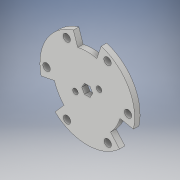
# Autodesk Inventor part: NewMechanumWheelHub
Saved by Autodesk Inventor 2017 (Build 210142000, 142)
## iProperties
Created: 2017-12-16
Part Number: NewMechanumWheelHub
Material: Generic
Document SubType Name: Modeling
Designer: User
Density: 1 g/cm^3
Appearance: Default
Author: User
Autodesk Inventor part; units mm, degrees
ref_plane "YZ Plane" through (0, 0, 0) normal (1, 0, 0) x (0, 1, 0)
ref_plane "XZ Plane" through (0, 0, 0) normal (0, 1, 0) x (-1, 0, 0)
ref_plane "XY Plane" through (0, 0, 0) normal (0, 0, 1) x (1, 0, 0)
sketch "Sketch1" plane through (0, 0, 0) normal (0, 0, 1) x (1, 0, 0)
  circle A0 centre (0, 0) radius 27.6352
  dimension "d0" = 55.2704
  constraints: 1 centre point, 1 coincident
  measures "d0" diameter of A0
extrude "Extrusion1" add sketch "Sketch1" along normal blind 3.175
sketch "Sketch2" plane through (0, 0, 3.175) normal (0, 0, 1) x (1, 0, 0)
  circle A0 centre (0, 0) radius 27.6352 projected
  line L0 (0, 27.6352) -> (0, 0)
  line L1 (0, 0) -> (23.9328, -13.8176)
  line L2 (0, 0) -> (-23.9328, -13.8176)
  line L3 (0, 0) -> (27.6352, 0) construction
  line L4 (0, 27.6352) -> (0, 19.4152)
  line L5 (0, 19.4152) -> (5.08, 19.4152)
  line L6 (0, 19.4152) -> (-5.08, 19.4152)
  arc A1 (5.08, 19.4152) -> (-5.08, 19.4152) centre (0, -5.5937) ccw
  line L7 (-5.08, 19.4152) -> (2.5298, 19.4152) construction
  line L8 (-5.08, 19.4152) -> (-7.5281, 26.5901)
  line L9 (-5.08, 19.4152) -> (2.501, 19.4152) construction
  line L10 (5.08, 19.4152) -> (7.5281, 26.5901)
  line L11 (5.08, 19.4152) -> (12.661, 19.4152) construction
  line L12 (23.9328, -13.8176) -> (16.8277, -9.7155)
  line L13 (16.8277, -9.7155) -> (19.355, -5.3381)
  line L14 (16.8277, -9.7155) -> (14.3004, -14.0929)
  line L15 (16.8277, -9.7155) -> (17.2897, -9.9822)
  arc A2 (14.3004, -14.0929) -> (19.355, -5.3381) centre (-3.6819, 2.1257) ccw
  point P0 (0.3732, 19.9232)
  point P1 (0, 19.9259)
  dimension "d3" = 120
  dimension "d5" = 120
  dimension "d6" = 120
  dimension "d7" = 8.22
  dimension "d8" = 5.08
  dimension "d9" = 5.08
  dimension "d11" = 108.84
  dimension "d12" = 71.16
  dimension "d13" = 8.2042
  dimension "d14" = 5.0546
  dimension "d15" = 5.0546
  dimension "d16" = 6.16
  dimension "d17" = 0.5334
  dimension "d51" = 0.508
  constraints: 32 end point, 12 point on circle, 6 horizontal, 3 equal length, 3 point on line, 2 centre point, 2 coincident, 1 perpendicular, 1 vertical
  measures "d3" angle of L1 L0
  measures "d5" angle of L0 L2
  measures "d6" angle of L2 L1
  measures "d7" distance of L0.start L4.end
  measures "d8" distance of L4.end L5.end
  measures "d9" distance of L4.end L6.end
  measures "d11" angle of L9 L8
  measures "d12" angle of L11 L10
  measures "d13" distance of L1.end L12.end
  measures "d14" distance of L12.end L13.end
  measures "d15" distance of L12.end L14.end
  measures "d17" distance of L12.end L15.end
  measures "d51" distance from line of L6 point (0.373, 19.923)
extrude "Extrusion2" cut sketch "Sketch2" against normal blind 3.175 contours L10 A1 L0 A0 | L0 A1 L8 A0
pattern_circular "Circular Pattern1" count 3 over 360 about axis through (0, 0, 0) along (0, 0, 1) of "Extrusion2"
sketch "Sketch4" plane through (0, 0, 3.175) normal (0, 0, 1) x (1, 0, 0)
  line L0 (-1.6129, 2.7686) -> (1.6129, 2.7686)
  line L1 (-1.6129, -2.7686) -> (1.6129, -2.7686)
  line L2 (0, 2.7686) -> (0, 0)
  line L3 (0, -2.7686) -> (0, 0)
  line L4 (-1.6129, 2.7686) -> (1.5912, 2.7811)
  line L5 (1.5912, 2.7811) -> (3.2041, 0.0125)
  line L6 (3.2041, 0.0125) -> (1.6129, -2.7686)
  line L7 (1.6129, -2.7686) -> (-1.5912, -2.7811)
  line L8 (-1.5912, -2.7811) -> (-3.2041, -0.0125)
  line L9 (-3.2041, -0.0125) -> (-1.6129, 2.7686)
  constraints: 20 end point, 2 horizontal, 2 midpoint, 2 vertical, 1 coincident, 13 other
extrude "Extrusion3" cut sketch "Sketch4" against normal blind 25.4
sketch "Sketch5" plane through (0, 0, 3.175) normal (0, 0, 1) x (1, 0, 0)
  line L0 (0, 0) -> (-11.9711, 20.5846)
  line L1 (-5.08, 19.4152) -> (-7.5281, 26.5901) projected
  circle A0 centre (-11.9711, 20.5846) radius 2.159
  line L2 (0, 0) -> (11.8412, 20.6596)
  line L3 (7.5281, 26.5901) -> (5.08, 19.4152) projected
  circle A1 centre (11.8412, 20.6596) radius 2.159
  line L4 (0, 0) -> (23.8124, 0.075)
  line L5 (19.3541, -5.3082) -> (26.7917, -6.7755) projected
  circle A2 centre (23.8124, 0.075) radius 2.159
  line L6 (0, 0) -> (11.9959, -20.5702)
  line L7 (19.2636, -19.8146) -> (14.2741, -14.107) projected
  circle A3 centre (11.9959, -20.5702) radius 2.159
  line L8 (0, 0) -> (-11.8291, -20.6666)
  line L9 (-14.2741, -14.107) -> (-19.2636, -19.8146) projected
  circle A4 centre (-11.8291, -20.6666) radius 2.159
  line L10 (-19.3541, -5.3082) -> (-26.7917, -6.7755) projected
  line L11 (0, 0) -> (-23.7488, -0.1036)
  line L12 (0, 0) -> (23.749, 0) construction
  dimension "d52" = 23.8125
  dimension "d54" = 4.318
  dimension "d55" = 23.8125
  dimension "d57" = 4.318
  dimension "d58" = 23.8125
  dimension "d60" = 4.318
  dimension "d61" = 23.8125
  dimension "d63" = 4.318
  dimension "d64" = 23.8125
  dimension "d66" = 4.318
  dimension "d69" = 23.8125
  dimension "d70" = 23.8252
  dimension "d82" = 5.969
  dimension "d86" = 59.931
  dimension "d88" = 23.749
  dimension "d89" = 180.25
  constraints: 14 end point, 6 coincident, 5 centre point, 1 equal length, 1 horizontal
  measures "d52" distance of L0.start L0.end
  measures "d54" diameter of A0
  measures "d55" distance of L0.start L2.end
  measures "d57" diameter of A1
  measures "d58" distance of L0.start L4.end
  measures "d60" diameter of A2
  measures "d61" distance of L0.start L6.end
  measures "d63" diameter of A3
  measures "d64" distance of L0.start L8.end
  measures "d66" diameter of A4
  measures "d69" distance of L2.end L0.end
  measures "d70" distance of L6.end L8.end
  measures "d82" distance from line of L7 L6.end
  measures "d86" angle of L4 L6
  measures "d88" distance of L0.start L11.end
extrude "Extrusion4" cut sketch "Sketch5" against normal blind 25.4
hole "Hole2" at (-23.7488, -0.1036, 3.175) direction (0, 0, -1) diameter 4.318 depth 25.4 tip angle 118
sketch "Sketch7" plane through (0, 0, 3.175) normal (0, 0, 1) x (1, 0, 0)
  line L0 (1.5912, 2.7811) -> (3.2041, 0.0125) projected
  line L1 (2.3977, 1.3968) -> (6.897, 4.0176)
  line L2 (2.3977, 1.3968) -> (7.6047, 1.3968) construction
  circle A0 centre (6.897, 4.0176) radius 1.5875
  point P0 (0, 0)
  dimension "d105" = 5.207
  dimension "d106" = 30.22
  dimension "d107" = 3.175
  constraints: 4 end point, 1 centre point, 1 coincident, 1 equal length, 1 horizontal, 1 midpoint
  measures "d105" distance of L1.start L1.end
  measures "d106" angle of L2 L1
  measures "d107" diameter of A0
extrude "Extrusion5" cut sketch "Sketch7" against normal blind 25.4
sketch "Sketch8" plane through (0, 0, 3.175) normal (0, 0, 1) x (1, 0, 0)
  line L0 (-3.2041, -0.0125) -> (-1.5912, -2.7811) projected
  line L1 (-2.3977, -1.3968) -> (-6.8969, -4.0179)
  circle A0 centre (-6.8969, -4.0179) radius 1.5875
  point P0 (0, 0)
  dimension "d112" = 5.207
  dimension "d113" = 3.175
  constraints: 2 end point, 1 centre point, 1 coincident, 1 midpoint
  measures "d112" distance of L1.start L1.end
  measures "d113" diameter of A0
extrude "Extrusion6" cut sketch "Sketch8" against normal blind 25.4
thicken "Thicken1" operation add thickness 0.635 both sides no extend neighbours yes toward (-0.946424, -0.3229265, 0) faces at (-6.7121, 24.1984, 1.0583)
thicken "Thicken2" operation add thickness 0.635 both sides no extend neighbours yes toward (0.946424, -0.3229265, 0) faces at (5.896, 21.8068, 2.1167)
thicken "Thicken3" operation add thickness 0.635 both sides no extend neighbours yes toward (0.1935495, 0.9810905, 0) faces at (24.3125, -6.2864, 2.1167)
thicken "Thicken4" operation add thickness 0.635 both sides no extend neighbours yes toward (-0.7528746, -0.658164, 0) faces at (17.6004, -17.9121, 1.0583)
thicken "Thicken5" operation add thickness 0.635 both sides no extend neighbours yes toward (-0.1935495, 0.9810905, 0) faces at (-21.8333, -5.7973, 2.1167)
thicken "Thicken6" operation add thickness 0.635 both sides no extend neighbours yes toward (0.7528746, -0.658164, 0) faces at (-17.6004, -17.9121, 2.1167)
thicken "Thicken7" operation add thickness 0.381 both sides no extend neighbours yes toward (0.1744546, -0.9846652, 0) faces at (-4.452, 19.5346, 2.1167)
thicken "Thicken8" operation add thickness 0.381 both sides no extend neighbours yes toward (-0.9217033, 0.3878957, 0) faces at (18.6772, -7.1021, 1.0583)
thicken "Thicken9" operation add thickness 0.381 both sides no extend neighbours yes toward (0.7655178, 0.6434147, 0) faces at (-14.6914, -13.6229, 2.1167)
equation "\"d55\" = d52"
equation "\"d58\" = d52"
equation "\"d61\" = d52"
equation "\"d64\" = d52"
equation "\"d69\" = d52"
body "Solid1"
